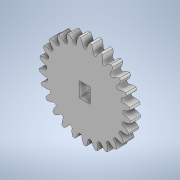
# Autodesk Inventor part: Pinion Real
Saved by Autodesk Inventor 2020 (Build 240168000, 168)
## iProperties
Created: 2020-11-24
Part Number: Pinion Real
Material: Generic
Document SubType Name: Modeling
Designer: shaun
Density: 1 g/cm^3
Appearance: Default
Author: shaun
Autodesk Inventor part; units mm, degrees
ref_plane "YZ Plane" through (0, 0, 0) normal (1, 0, 0) x (0, 1, 0)
ref_plane "XZ Plane" through (0, 0, 0) normal (0, 1, 0) x (-1, 0, 0)
ref_plane "XY Plane" through (0, 0, 0) normal (0, 0, 1) x (1, 0, 0)
sketch "Sketch1" plane through (0, 0, 0) normal (0, 0, 1) x (1, 0, 0)
  spline S0 degree 3 poles (-1.3621, 13.5316) (-1.3292, 13.4857) (-1.2634, 13.394) (-1.1694, 13.2531) (-1.0789, 13.11) (-0.9926, 12.9642) (-0.9108, 12.816) (-0.8338, 12.6651) (-0.7622, 12.5116) (-0.6965, 12.3555) (-0.6377, 12.1967) (-0.5868, 12.0351) (-0.5531, 11.898) (-0.533, 11.7869) (-0.5104, 11.7051) (-0.4797, 11.6261) (-0.4449, 11.5644) (-0.4127, 11.518) (-0.3847, 11.4862) (-0.355, 11.4559) (-0.3216, 11.4298) (-0.2867, 11.4058) (-0.2487, 11.3868) (-0.2098, 11.37) (-0.1686, 11.36) (-0.1271, 11.3512) (-0.0705, 11.3492) (0, 11.3505) (0.0705, 11.3492) (0.1271, 11.3512) (0.1686, 11.36) (0.2098, 11.37) (0.2487, 11.3868) (0.2867, 11.4058) (0.3216, 11.4298) (0.355, 11.4559) (0.3847, 11.4862) (0.4127, 11.518) (0.4449, 11.5644) (0.4797, 11.6261) (0.5104, 11.7051) (0.533, 11.7869) (0.5531, 11.898) (0.5868, 12.0351) (0.6377, 12.1967) (0.6965, 12.3555) (0.7622, 12.5116) (0.8338, 12.6651) (0.9108, 12.816) (0.9926, 12.9642) (1.0789, 13.11) (1.1694, 13.2531) (1.2634, 13.394) (1.3292, 13.4857) (1.3621, 13.5316) knots 0 0 0 0 0.016933 0.033866 0.0508 0.067733 0.084666 0.101599 0.118531 0.135464 0.152396 0.169328 0.186257 0.194723 0.203188 0.211652 0.220111 0.224346 0.228579 0.232811 0.237045 0.241276 0.245509 0.249742 0.253974 0.258206 0.262439 0.270905 0.279372 0.283605 0.287836 0.292069 0.296302 0.300535 0.304766 0.309 0.313231 0.317465 0.3217 0.330159 0.338623 0.347088 0.355554 0.372483 0.389415 0.406347 0.423279 0.440212 0.457145 0.474078 0.491011 0.507944 0.524878 0.541811 0.541811 0.541811 0.541811
  circle A0 centre (0, 0) radius 11.35 construction
  circle A1 centre (0, 0) radius 11.7462 construction
  circle A2 centre (0, 0) radius 12.5 construction
  circle A3 centre (0, 0) radius 13.6
  point P0 (-1.2642, 13.3934)
  point P1 (-1.17, 13.2527)
  point P2 (-1.0796, 13.1095)
  point P3 (-0.9933, 12.9638)
  point P4 (-0.9116, 12.8155)
  point P5 (-0.8347, 12.6647)
  point P6 (-0.7632, 12.5112)
  point P7 (-0.6976, 12.3551)
  point P8 (-0.639, 12.1962)
  point P9 (-0.5886, 12.0346)
  point P10 (-0.5486, 11.8701)
  point P11 (-0.5317, 11.7871)
  point P12 (-0.509, 11.7056)
  point P13 (-0.4778, 11.6269)
  point P14 (-0.4365, 11.5531)
  point P15 (-0.4121, 11.5185)
  point P16 (-0.3844, 11.4864)
  point P17 (-0.3544, 11.4566)
  point P18 (-0.3214, 11.4301)
  point P19 (-0.2862, 11.4066)
  point P20 (-0.2486, 11.3872)
  point P21 (-0.2094, 11.3711)
  point P22 (-0.1685, 11.3602)
  point P23 (-0.1269, 11.3524)
  point P24 (-0.0847, 11.35)
  point P25 (0, 11.35)
  point P26 (0.0847, 11.35)
  point P27 (0.1269, 11.3524)
  point P28 (0.1685, 11.3602)
  point P29 (0.2094, 11.3711)
  point P30 (0.2486, 11.3872)
  point P31 (0.2862, 11.4066)
  point P32 (0.3214, 11.4301)
  point P33 (0.3544, 11.4566)
  point P34 (0.3844, 11.4864)
  point P35 (0.4121, 11.5185)
  point P36 (0.4365, 11.5531)
  point P37 (0.4778, 11.6269)
  point P38 (0.509, 11.7056)
  point P39 (0.5317, 11.7871)
  point P40 (0.5486, 11.8701)
  point P41 (0.5886, 12.0346)
  point P42 (0.639, 12.1962)
  point P43 (0.6976, 12.3551)
  point P44 (0.7632, 12.5112)
  point P45 (0.8347, 12.6647)
  point P46 (0.9116, 12.8155)
  point P47 (0.9933, 12.9638)
  point P48 (1.0796, 13.1095)
  point P49 (1.17, 13.2527)
  point P50 (1.2642, 13.3934)
  constraints: 4 centre point, 2 point on circle, 111 other
extrude "Extrusion1" add sketch "Sketch1" against normal blind 3
extrude "Extrusion2" cut sketch "Sketch1" against normal blind 10 contours A3 S0 picked at (-0.1392, 12.8204)
pattern_circular "Circular Pattern1" count 25 over 360 about axis through (0, 0, -10) along (0, 0, 1) of "Extrusion2"
sketch "Sketch2" plane through (0, 0, 0) normal (0, 0, 1) x (1, 0, 0)
  line L0 (-1.6041, 2.298) -> (1.5959, 2.298)
  line L1 (1.5959, 2.298) -> (1.5959, -2.102)
  line L2 (1.5959, -2.102) -> (-1.6041, -2.102)
  line L3 (-1.6041, -2.102) -> (-1.6041, 2.298)
  point P0 (0, 0)
  point P1 (0, 0)
  point P2 (0.0017, -0.002)
  dimension "d10" = 4.4
  dimension "d11" = 3.2
  constraints: 8 end point, 2 parallel, 1 coincident, 1 horizontal, 1 perpendicular
  measures "d10" distance between parallel lines of L2 L0
  measures "d11" distance between parallel lines of L1 L3
extrude "Extrusion3" cut sketch "Sketch2" against normal blind 10
equation "\"Module\" = 1"
equation "\"PressureAngle\" = 20deg"
equation "\"UnitProfileClearance\" = 0.25"
equation "\"UnitRoundRadius\" = 0.35"
equation "\"HeadDiameter\" = 27.2"
equation "\"RootDiameter\" = 22.7"
equation "\"BaseDiameter\" = 23.49232"
equation "\"PitchDiameter\" = 25"
equation "\"FaceWidth\" = 3"
equation "\"HelixAngle\" = 0"
equation "\"UnitCorrection\" = 0.1"
equation "\"UnitAddendumModification\" = 0"
equation "\"CircularPitch\" = 3.141593"
equation "\"UnitBacklashShift\" = 0"
equation "\"TotalToolShift\" = 0.1"
equation "\"IsInternal\" = 0"
body "Solid1"
